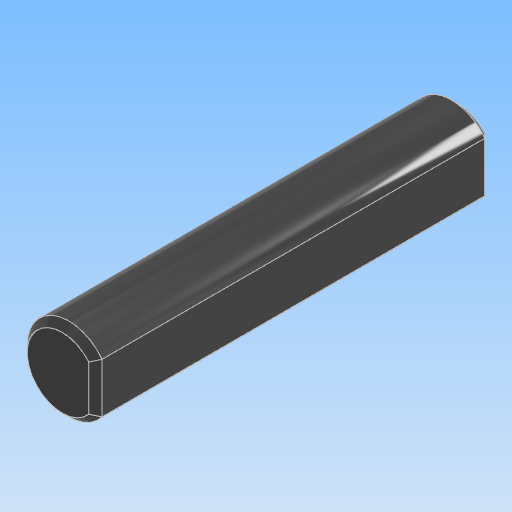
# Autodesk Inventor part: V1_Cycloid_Cam
Saved by Autodesk Inventor 2021 (Build 250183000, 183)
## iProperties
Created: 2020-12-17
Part Number: V1_Cycloid_Cam
Material: PPS Plastic
Document SubType Name: Modeling
Designer: ndevr
Density: 1.637 g/cm^3
Appearance: Smooth - White
Spacer:Thick: 0.008 in
Author: ndevr
Autodesk Inventor part; units mm, degrees
ref_plane "YZ Vertical Spine" through (0, 0, 0) normal (1, 0, 0) x (0, 1, 0)
ref_plane "XZ Vertical Span" through (0, 0, 0) normal (0, 1, 0) x (-1, 0, 0)
sketch "Nema 23 Mount" plane through (0, 0, 0) normal (0, 0, 1) x (1, 0, 0)
  circle A0 centre (-8.8943, 7.749) radius 1.5
  circle A1 centre (22.1057, 7.749) radius 1.5
  line L0 (-8.8943, 7.749) -> (22.1057, 7.749) construction
  line L1 (22.1057, 7.749) -> (22.1057, -23.251) construction
  line L2 (22.1057, -23.251) -> (-8.8943, -23.251) construction
  line L3 (-8.8943, -23.251) -> (-8.8943, 7.749) construction
  circle A2 centre (-8.8943, -23.251) radius 1.5
  circle A3 centre (22.1057, -23.251) radius 1.5
  line L4 (-8.8943, 7.749) -> (22.1057, -23.251) construction
  dimension "d67" = 31
  dimension "d68" = 3
  measures "d67" distance of L2.end L0.start
  measures "d68" diameter of A2
derived "V1_N17Cycloid_Geo.ipt"
sketch "Cycloid.sk" plane through (0, 0, 0) normal (0, 0, 1) x (1, 0, 0)
  spline S0 degree 3 number of poles 685
  point P0 (30.7397, 0)
  point P1 (0, 0)
sketch "Cycloid Gear.sk" plane through (0, 0, 0) normal (0, 0, 1) x (1, 0, 0)
  circle A0 centre (20.862, 0) radius 3.4365
  circle A1 centre (0, 0) radius 6.7333
  circle A2 centre (21.9203, 0) radius 4.5583
  circle A3 centre (0, 21.9203) radius 4.5583
  circle A4 centre (-21.9203, 0) radius 4.5583
  circle A5 centre (0, -21.9203) radius 4.5583
  spline S0 degree 3 number of poles 685
  circle A6 centre (-1.0583, 0) radius 2.5
  line L0 (0.9417, 1.5) -> (0.9417, -1.5)
  circle A7 centre (-1.0583, 21.9203) radius 1.5
  circle A8 centre (20.862, 0) radius 1.5
  line L1 (-1.0583, 21.9203) -> (20.862, 0) construction
  line L2 (20.862, 0) -> (-1.0583, -21.9203) construction
  line L3 (-1.0583, -21.9203) -> (-22.9786, 0) construction
  line L4 (-22.9786, 0) -> (-1.0583, 21.9203) construction
  circle A9 centre (-22.9786, 0) radius 1.5
  circle A10 centre (-1.0583, -21.9203) radius 1.5
  line L5 (-1.0583, 21.9203) -> (-1.0583, -21.9203) construction
  point P0 (41.275, 0)
  point P1 (-2.1167, 0)
sketch "Rollers.sk" plane through (0, 0, 0) normal (0, 0, 1) x (1, 0, 0)
  circle A0 centre (33.8667, 0) radius 3.0635
  circle A1 centre (32.6766, 9.0393) radius 3.0635
  circle A2 centre (29.1876, 17.4625) radius 3.0635
  circle A3 centre (23.6374, 24.6957) radius 3.0635
  circle A4 centre (16.4042, 30.2459) radius 3.0635
  circle A5 centre (7.9809, 33.735) radius 3.0635
  circle A6 centre (-1.0583, 34.925) radius 3.0635
  circle A7 centre (-10.0976, 33.735) radius 3.0635
  circle A8 centre (33.8667, 0) radius 3.127 construction
  circle A9 centre (-18.5208, 30.2459) radius 3.0635
  circle A10 centre (-25.754, 24.6957) radius 3.0635
  circle A11 centre (-31.3043, 17.4625) radius 3.0635
  circle A12 centre (-34.7933, 9.0393) radius 3.0635
  circle A13 centre (-35.9833, 0) radius 3.0635
  circle A14 centre (-34.7933, -9.0393) radius 3.0635
  circle A15 centre (-31.3043, -17.4625) radius 3.0635
  circle A16 centre (-25.754, -24.6957) radius 3.0635
  circle A17 centre (-18.5208, -30.2459) radius 3.0635
  circle A18 centre (-10.0976, -33.735) radius 3.0635
  circle A19 centre (-1.0583, -34.925) radius 3.0635
  circle A20 centre (7.9809, -33.735) radius 3.0635
  circle A21 centre (16.4042, -30.2459) radius 3.0635
  circle A22 centre (23.6374, -24.6957) radius 3.0635
  circle A23 centre (29.1876, -17.4625) radius 3.0635
  circle A24 centre (32.6766, -9.0393) radius 3.0635
  point P0 (0, 0)
  point P1 (-1.0583, 0)
ref_plane "Top Output Top" through (9.525, 0, 19.05) normal (0, 0, -1) x (-1, 0, 0)
ref_plane "Bot Cycoid Top" through (9.525, 0, 16.8672) normal (0, 0, -1) x (-1, 0, 0)
ref_plane "Bot Cycoid Bot" through (9.525, 0, 10.5172) normal (0, 0, -1) x (-1, 0, 0)
ref_plane "Bot Output Top" through (9.525, 0, 10.3188) normal (0, 0, -1) x (-1, 0, 0)
ref_plane "Bot Output Bot" through (9.525, 0, 1.5875) normal (0, 0, -1) x (-1, 0, 0)
ref_plane "Top Cycloid Top" through (9.525, 0, 23.6141) normal (0, 0, -1) x (-1, 0, 0)
ref_plane "Top Cycloid Bot" through (9.525, 0, 17.2641) normal (0, 0, -1) x (-1, 0, 0)
sketch "Sketch16" plane through (0, 0, 0) normal (0, 0, 1) x (1, 0, 0)
  circle A0 centre (0, 0) radius 6.7333 construction
  circle A1 centre (0, 0) radius 6.7333
  circle A2 centre (-1.0583, 0) radius 2.5 projected
  line L0 (0.9417, 1.5) -> (0.9417, -1.5) projected
  circle A3 centre (-1.0583, 0) radius 2.6016
  line L1 (1.0433, 1.5335) -> (1.0433, -1.5335)
  dimension "d88" = 0
  dimension "d89" = 0.1016
  dimension "d90" = 0.1016
  constraints: 2 centre point, 2 coincident, 2 end point, 2 point on circle, 1 parallel
  measures "d88" radial gap between concentric circles of A0 A1
  measures "d89" distance between parallel lines of L1 L0
  measures "d90" radial gap between concentric circles of A3 A2
ref_plane "Work Plane19" through (9.525, 0, 25.4) normal (0, 0, -1) x (-1, 0, 0)
extrude "Extrusion13" add sketch "Sketch16" along normal up to surface (23.8125 mm away) from surface at 1.5875 contours L0 A2
chamfer "Chamfer8" distance 0.3969 angle 45 4 edges at (-3.5583, 0, 25.4) (-3.5583, 0, 1.5875) (0.9417, 0, 25.4) (0.9417, 0, 1.5875)
equation "\"d90\" = d89"
body "Solid6"
